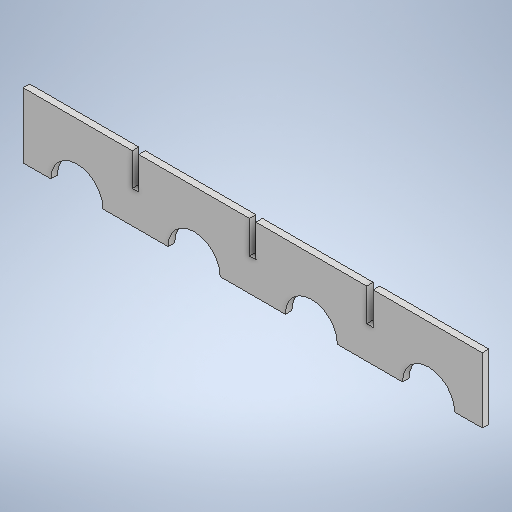
# Autodesk Inventor part: BSH 085 amplifier bottom
Saved by Autodesk Inventor 2025 (Build 290162010, 162A)
## iProperties
Created: 2024-08-04
Part Number: BSH 085 amplifier bottom
Material: Stainless Steel
Document SubType Name: Sheet Metal
Designer: pokla
Density: 8 g/cm^3
Sheet Metal Rule: AISI304 2mm Die16
Appearance: Default
Author: pokla
Autodesk Inventor part; units mm, degrees
ref_plane "YZ Plane" through (0, 0, 0) normal (1, 0, 0) x (0, 1, 0)
ref_plane "XZ Plane" through (0, 0, 0) normal (0, 1, 0) x (-1, 0, 0)
ref_plane "XY Plane" through (0, 0, 0) normal (0, 0, 1) x (1, 0, 0)
sketch "Sketch1" plane through (0, 0, 0) normal (0, 0, 1) x (1, 0, 0)
  circle A0 centre (0, 0) radius 400 construction
  line L0 (-352.5, 175) -> (352.5, 175)
  line L1 (352.5, 175) -> (352.5, 185)
  line L2 (352.5, 185) -> (-352.5, 185)
  line L3 (-352.5, 185) -> (-352.5, 175)
  line L4 (-352.5, 185) -> (352.5, 175) construction
  point P0 (0, 180)
  dimension "d0" = 800
  dimension "d24" = 10
  dimension "d25" = 180
  dimension "d26" = 705
  constraints: 10 end point, 3 coincident, 2 parallel, 1 centre point, 1 horizontal, 1 midpoint, 1 perpendicular, 1 vertical alignment
  measures "d0" diameter of A0
  measures "d24" distance of L2.end L0.start
  measures "d25" distance of point (0, 180) point (0, 0)
  measures "d26" distance of L1.end L2.end
extrude "Extrusion1" add sketch "Sketch1" along normal blind 100
sketch "Sketch3" plane through (-352.5, 175, 0) normal (0, -1, 0) x (1, 0, 0)
  line L0 (705, 0) -> (0, 0) projected
  circle A0 centre (82.5, 0) radius 40
  circle A1 centre (262.5, 0) radius 40
  circle A2 centre (442.5, 0) radius 40
  line L1 (0, 0) -> (705, 0) projected
  circle A3 centre (622.5, 0) radius 40
  line L2 (347.5, 100) -> (357.5, 100)
  line L3 (357.5, 100) -> (357.5, 50)
  line L4 (357.5, 50) -> (347.5, 50)
  line L5 (347.5, 50) -> (347.5, 100)
  line L6 (0, 100) -> (705, 100) projected
  line L7 (167.5, 100) -> (177.5, 100)
  line L8 (177.5, 100) -> (177.5, 50)
  line L9 (177.5, 50) -> (167.5, 50)
  line L10 (167.5, 50) -> (167.5, 100)
  line L11 (527.5, 100) -> (537.5, 100)
  line L12 (537.5, 100) -> (537.5, 50)
  line L13 (537.5, 50) -> (527.5, 50)
  line L14 (527.5, 50) -> (527.5, 100)
  point P0 (352.5, 0)
  point P1 (352.5, 0)
  point P2 (352.5, 100)
  point P3 (352.5, 100)
  point P4 (352.5, 100)
  point P5 (172.5, 100)
  point P6 (352.5, 100)
  point P7 (352.5, 100)
  point P8 (532.5, 100)
  point P9 (352.5, 100)
  point P10 (352.5, 100)
  point P11 (42.5, 0)
  point P12 (122.5, 0)
  point P13 (222.5, 0)
  point P14 (302.5, 0)
  point P15 (402.5, 0)
  point P16 (482.5, 0)
  point P17 (582.5, 0)
  point P18 (662.5, 0)
  dimension "d59" = 80
  dimension "d60" = 80
  dimension "d61" = 90
  dimension "d62" = 180
  dimension "d63" = 80
  dimension "d64" = 90
  dimension "d65" = 80
  dimension "d66" = 180
  dimension "d67" = 10
  dimension "d68" = 50
  dimension "d69" = 180
  dimension "d70" = 10
  dimension "d71" = 50
  dimension "d72" = 180
  dimension "d73" = 50
  dimension "d74" = 10
  constraints: 24 end point, 11 midpoint, 6 parallel, 4 centre point, 4 point on line, 3 horizontal, 3 perpendicular, 2 coincident, 2 horizontal alignment
  measures "d59" diameter of A0
  measures "d60" diameter of A1
  measures "d61" distance of point (352.5, 0) A1.centre
  measures "d62" distance of A0.centre A1.centre
  measures "d63" diameter of A2
  measures "d64" distance of point (352.5, 0) A2.centre
  measures "d65" diameter of A3
  measures "d66" distance of A2.centre A3.centre
  measures "d67" distance between parallel lines of L5 L3
  measures "d68" distance of L4.end L2.start
  measures "d69" distance of point (352.5, 100) point (172.5, 100)
  measures "d70" distance between parallel lines of L10 L8
  measures "d71" distance of L9.end L7.start
  measures "d72" distance of point (352.5, 100) point (532.5, 100)
  measures "d73" distance of L13.end L11.start
  measures "d74" distance between parallel lines of L14 L12
extrude "Extrusion3" cut sketch "Sketch3" against normal through all contours L0 A3 | L0 A2 | L0 A1 | L0 A0 | L2 L3 L4 L5 | L6 L8 L9 L10 | L6 L12 L13 L14 picked at (611.7131, 7.8371) picked at (435.8333, 20.5179) picked at (255.8333, 20.5179) picked at (84.0738, 20.5179)
equation "\"d70\" = d67"
equation "\"d71\" = d68"
equation "\"BendReliefWidth\" = Thickness"
equation "\"BendReliefDepth\" = 0.5 * Thickness"
equation "\"CornerReliefSize\" = 4 * Thickness"
equation "\"MinimumRemnant\" = 2 * Thickness"
equation "\"TransitionRadius\" = BendRadius"
equation "\"JacobiRadiusSize\" = BendRadius"
equation "\"GapSize\" = Thickness"
equation "\"Thickness\" = 2"
equation "\"BendRadius\" = 2.75"
body "Solid1"
